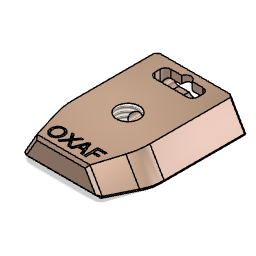
specimen puck v19 (Autodesk Fusion 360 design; units mm, degrees)
Autodesk Fusion 360 part; units mm, degrees
note: some values were not read from the file. Chosen so that the rebuilt part matches the saved one: which face or edge a step refers to; the sign of a taper; which pieces of a blend or face edit are solid. Set by a fixed rule: which sketch regions a step uses; the direction of a hole.
sketch "Sketch1" plane through (0, 0, 0) normal (0, 0, 1) x (1, 0, 0)
  line L0 (10, 0) -> (-10, 0)
  line L1 (-10, 0) -> (-7.1132, 5)
  line L2 (-7.1132, 5) -> (7.1132, 5)
  line L3 (7.1132, 5) -> (10, 0)
  line L4 (0, 2.5) -> (0, 20)
  line L5 (-8.5566, 2.5) -> (8.5566, 2.5) construction
  line L6 (4, 3.5) -> (4, 1.5)
  line L7 (4, 3.5) -> (-4, 3.5)
  line L8 (-4, 3.5) -> (-4, 1.5)
  line L9 (-4, 1.5) -> (4, 1.5)
  dimension "d1" = 20
  dimension "d2" = 5
  dimension "d3" = 60
  dimension "d5" = 8
  dimension "d7" = 2
  constraint horizontal L0
  constraint parallel L0 L2
  constraint coincident origin L0
  constraint symmetric L1 L3 L4
  constraint midpoint L1 L5.start
  constraint midpoint L3 L5.end
  constraint perpendicular L5 L6
  constraint parallel L5 L7
  constraint perpendicular L5 L8
  constraint perpendicular L8 L9
  constraint symmetric L4 L6 L8
  constraint coincident L6.start L7.start
  constraint coincident L6.end L9.end
  constraint symmetric L5 L7 L9
  measures "d1" distance of L0.start L0.end
  measures "d2" distance of L0 L2
  measures "d3" angle of L1 L3
  measures "d5" distance of L6 L8
  measures "d7" distance of L7 L9
extrude "Extrude1" add sketch "Sketch1" along normal blind 25 contours L0 L1 L2 L3 | L6 L7 L8 L9
sketch "Sketch2" plane through (0, 0, 0) normal (0, 1, 0) x (1, 0, 0)
  line L0 (-4, -4.5) -> (4, -4.5)
  line L1 (4, -4.5) -> (4, -1.5)
  line L2 (4, -1.5) -> (-4, -1.5)
  line L3 (-4, -1.5) -> (-4, -4.5)
  line L4 (10, 0) -> (-10, 0)
  line L5 (0, -1.75) -> (0, -22.5)
  point P0 (-4, 0)
  point P1 (4, 0)
  point P2 (0, -1.75)
  point P3 (0, -12.5)
  dimension "d10" = 3
  dimension "d11" = 1.5
  dimension "d27" = 12.5
  dimension "d42" = 0.25
  constraint horizontal L0
  constraint vertical L1
  constraint horizontal L2
  constraint vertical L3
  constraint coincident L1 P1
  constraint coincident L3 P0
  constraint coincident L5 P3
  constraint coincident L5 P2
  measures "d10" distance of L0 L2
  measures "d11" distance of L2 L4
  measures "d27" distance of origin P3
  measures "d42" distance of L2 P2
sketch "Sketch3" plane through (0, 5, 0) normal (0, 1, 0) x (-1, 0, 0)
  line L0 (-7.1132, 0) -> (7.1132, 0)
  line L1 (7.1132, 0) -> (7.1132, 25)
  line L2 (7.1132, 25) -> (-7.1132, 25)
  line L3 (-7.1132, 25) -> (-7.1132, 0)
  point P0 (0, 12.5)
hole "Hole1" at (0, 2.5, 0) direction (0, 0, 1) diameter 3 depth 12 tip angle 118
hole "Hole2" at (0, 0, 1.75) direction (0, 1, 0) diameter 2 end through all
extrude "Extrude2" cut sketch "Sketch1" along normal blind 3.5 contours L6 L7 L8 L9
extrude "Extrude3" cut sketch "Sketch2" along normal through all
ref_plane "WorkPlane1" through (0, 2.5, 17.5) normal (0, 0, 1) x (1, 0, 0)
split_face "SplitFace1" 3 faces at (8.0755, 3.3333, 8.3333) (-1.3333, 0, 18.1667) (-9.0377, 1.6667, 8.3333) by plane through (0, 2.5, 17.5) normal (0, 0, 1)
draft "Draft1" angle -15 neutral plane through (0, 2.5, 17.5) pull (0, 0, -1) 2 faces at (8.0755, 3.3333, 20) (-9.0377, 1.6667, 20)
draft "Draft2" angle -5 neutral plane through (0, 2.5, 17.5) pull (0, 0, -1) 1 faces at (-2.5598, 0, 20)
fillet "Fillet2" radius 15 2 edges at (8.5566, 2.5, 17.5) (-8.5566, 2.5, 17.5)
hole "Hole3" at (0, 5, 12.5) direction (0, -1, 0) diameter 4.234 end through all
thread "Thread1" "ISO Metric profile 5.0 M5x0.8 6H" thread offset 0 thread depth 10
chamfer "Chamfer1" distance 0.5 angle 45 14 edges at (0, 5, 25) (-6.0467, 2.8281, 25) (0, 0.6562, 25) (6.0467, 2.8281, 25) (8.3071, 0.4115, 22.2037) (9.6168, 0.084, 18.4599) (9.9623, 0, 16.5148) (10, 0, 7.7626) (8.5566, 2.5, 0) (-9.6168, 0.084, 18.4599) (-8.3071, 0.4115, 22.2037) (-10, 0, 7.7626) (-9.9623, 0, 16.5148) (-8.5566, 2.5, 0)
fillet "Fillet1" radius 1 10 edges at (-4, 2.5, 4.5) (-4, 4.25, 1.5) (-4, 0.75, 1.5) (4, 4.25, 1.5) (4, 0.75, 1.5) (4, 2.5, 4.5) (4, 1.5, 0.75) (4, 3.5, 0.75) (-4, 3.5, 0.75) (-4, 1.5, 0.75)
sketch "Skizze5" plane through (0, 5, 0) normal (0, 1, 0) x (-1, 0, 0)
  line L0 (3, 1.5) -> (0.9682, 1.5)
  arc A0 (-0.9682, 1.5) -> (0.9682, 1.5) centre (0, 1.75) ccw
  line L1 (-0.9682, 1.5) -> (-3, 1.5)
  arc A1 (-4, 2.5) -> (-3, 1.5) centre (-3, 2.5) ccw
  line L2 (-4, 2.5) -> (-4, 3.5)
  arc A2 (-3, 4.5) -> (-4, 3.5) centre (-3, 3.5) ccw
  line L3 (-3, 4.5) -> (3, 4.5)
  arc A3 (4, 3.5) -> (3, 4.5) centre (3, 3.5) ccw
  line L4 (4, 3.5) -> (4, 2.5)
  arc A4 (3, 1.5) -> (4, 2.5) centre (3, 2.5) ccw
  circle A5 centre (0, 12.5) radius 2.117
  line L5 (6.5359, 0) -> (7.1132, 0.5)
  line L6 (7.1132, 0.5) -> (7.1132, 15.5252)
  ellipse E0 centre (-10.2073, 15.5252) end of major axis (7.1132, 15.5252) minor radius 15 (7.1132, 15.5252) -> (6.5231, 19.4075) ccw
  line L7 (6.5231, 19.4075) -> (4.9474, 24.5)
  line L8 (4.9474, 24.5) -> (-4.9474, 24.5)
  line L9 (-4.9474, 24.5) -> (-6.5231, 19.4075)
  ellipse E1 centre (10.2073, 15.5252) end of major axis (-7.1132, 15.5252) minor radius 15 (-6.5231, 19.4075) -> (-7.1132, 15.5252) ccw
  line L10 (-7.1132, 15.5252) -> (-7.1132, 0.5)
  line L11 (-7.1132, 0.5) -> (-6.5359, 0)
  line L12 (-6.5359, 0) -> (6.5359, 0)
  line L13 (4.044, 23.5) -> (-3.956, 23.5406) construction
  line L14 (-3.956, 23.5406) -> (-3.9687, 21.0203) construction
  line L15 (-3.9687, 21.0203) -> (4.0312, 20.9798) construction
  line L16 (4.0312, 20.9798) -> (4.044, 23.5) construction
  dimension "d38" = 2.5
  dimension "d39" = 1
  text T0 "OXAF" font "Arial" height 2.5 align centre middle in box 8.0001 x 2.5203 at (4.044, 23.5) x (-0.999987, 0.005071) y (-0.005071, -0.999987) spacing 1
extrude "Extrusion4" cut sketch "Skizze5" against normal blind 0.5 text T0
chamfer "Chamfer2" [suppressed]
sketch "Sketch4" plane through (-3.5684, 6.1806, 0) normal (-0.5, 0.866025, 0) x (0, 0, 1)
  line L0 (0.5, -0.7265) -> (0.5, -4.5)
  line L1 (0.5, -4.5) -> (15.5252, -4.5)
  line L2 (15.5252, -4.5) -> (15.5252, -0.7265)
  line L3 (7, -4.8122) -> (14.5, -4.7942) construction
  line L4 (14.5, -4.7942) -> (14.4928, -1.7942) construction
  line L5 (14.4928, -1.7942) -> (6.9928, -1.8122) construction
  line L6 (6.9928, -1.8122) -> (7, -4.8122) construction
  line L7 (15.5252, -0.7265) -> (0.5, -0.7265)
  line L8 (0, -3.9593) -> (0.5, -4.9593)
  line L9 (0.5, -4.9593) -> (15.5252, -4.9593)
  line L10 (15.5252, -4.9593) -> (15.5252, -2.3612)
  line L11 (15.5252, -2.3612) -> (0, -2.3612)
  line L12 (0, -2.3612) -> (0, -3.9593)
  dimension "d34" = 7
  constraint perpendicular L3 L4
  constraint parallel L3 L5
  constraint parallel L4 L6
  measures "d34" horizontal distance of origin L3.start
